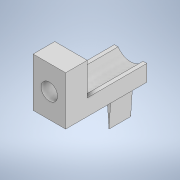
# Autodesk Inventor part: angle_pointer
Saved by Autodesk Inventor 2022 (Build 260153000, 153)
## iProperties
Created: 2021-03-02
Part Number: angle_pointer
Material: Generic
Document SubType Name: Modeling
Designer: dsdan
Density: 1 g/cm^3
Appearance: Default
Author: dsdan
Autodesk Inventor part; units mm, degrees
ref_plane "YZ Plane" through (0, 0, 0) normal (1, 0, 0) x (0, 1, 0)
ref_plane "XZ Plane" through (0, 0, 0) normal (0, 1, 0) x (-1, 0, 0)
ref_plane "XY Plane" through (0, 0, 0) normal (0, 0, 1) x (1, 0, 0)
sketch "Sketch1" plane through (0, 0, 0) normal (1, 0, 0) x (0, 1, 0)
  line L0 (0, 8) -> (0, 0)
  line L1 (0, 8) -> (15, 8)
  line L2 (15, 8) -> (15, 0)
  line L3 (6, 0) -> (6, 8) construction
  line L4 (0, 0) -> (15, 0)
  dimension "d38" = 6
  dimension "d40" = 8
  dimension "d59" = 15
  constraints: 10 end point, 2 horizontal, 2 perpendicular
  measures "d38" distance between parallel lines of L0 L3
  measures "d40" distance of L0.start L0.end
  measures "d59" distance of L0.start L1.end
extrude "Extrusion1" add sketch "Sketch1" along normal mid plane 12
sketch "Sketch3" plane through (6, 0, 8) normal (0, 0, 1) x (1, 0, 0)
  circle A0 centre (-6, 6) radius 3.05
  line L0 (-12, 0) -> (0, 0) projected
  line L1 (0, 15) -> (0, 0) projected
  point P0 (0, -6)
  point P1 (0, 12.26)
  dimension "d9" = 6.1
  dimension "d23" = 6
  dimension "d41" = 6
  constraints: 1 centre point, 1 other
  measures "d9" diameter of A0
  measures "d41" distance from line of L1 A0.centre
extrude "Extrusion3" cut sketch "Sketch3" against normal through all
sketch "Sketch8" plane through (-6, 0, 8) normal (0, 0, 1) x (1, 0, 0)
  circle A0 centre (6, 6) radius 3.05 construction
  circle A1 centre (6, 6) radius 5.5
  line L0 (0, 15) -> (0, 0) projected
  line L1 (0, 3) -> (1.3902, 3)
  line L2 (10.6098, 3) -> (12, 3)
  line L3 (12, 15) -> (12, 0) projected
  line L4 (12, 0) -> (12, -3)
  line L5 (12, -3) -> (0, -3)
  line L6 (0, -3) -> (0, 0)
  line L7 (0, 0) -> (12, 0) construction
  point P0 (6, 0)
  point P1 (12, 12.26)
  dimension "d47" = 11
  dimension "d48" = 6
  dimension "d49" = 3
  constraints: 10 end point, 4 point on line, 3 perpendicular, 2 point on circle, 1 centre point, 1 coincident, 1 vertical
  measures "d47" diameter of A1
  measures "d48" distance between parallel lines of L1 L5
  measures "d49" distance between parallel lines of L7 L1
extrude "Extrusion7" add sketch "Sketch8" against normal blind 30 contours A1 L2 L3 L4 L5 L6 L0 L1
sketch "Sketch9" plane through (-6, 0, -22) normal (0, 0, -1) x (-1, 0, 0)
  line L0 (-6.979, -3) -> (-6, -17)
  line L1 (-6, -17) -> (-5.021, -3)
  line L2 (-12, -3) -> (0, -3) projected
  line L3 (-6, -17) -> (-6, -3) construction
  point P0 (-6, 0)
  dimension "d54" = 14
  dimension "d55" = 4
  dimension "d56" = 4
  constraints: 6 end point, 3 point on line, 1 midpoint, 1 perpendicular
  measures "d54" distance from line of L2 L0.end
  measures "d55" angle of L0 L3
  measures "d56" angle of L1 L3
extrude "Extrusion8" add sketch "Sketch9" against normal blind 8
equation "\"d56\" = d55"
body "Solid1"
